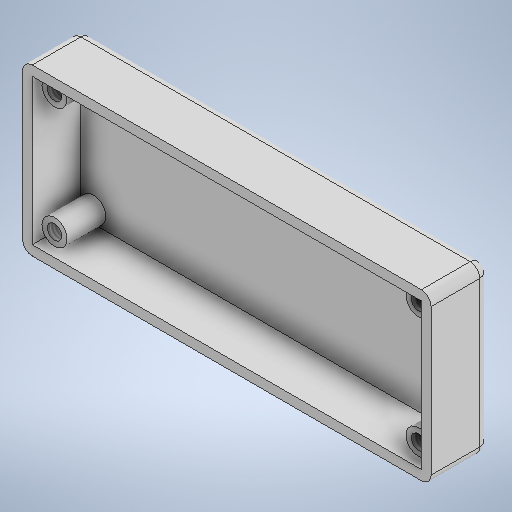
# Autodesk Inventor part: Bottom part of case
Saved by Autodesk Inventor 2025.2 (Build 292293000, 293)
## iProperties
Created: 2026-01-28
Part Number: Bottom part of case
Material: Generic
Document SubType Name: Modeling
Designer: seths
Density: 1 g/cm^3
Appearance: Default
Author: seths
Autodesk Inventor part; units mm, degrees
ref_plane "YZ Plane" through (0, 0, 0) normal (1, 0, 0) x (0, 1, 0)
ref_plane "XZ Plane" through (0, 0, 0) normal (0, 1, 0) x (-1, 0, 0)
ref_plane "XY Plane" through (0, 0, 0) normal (0, 0, 1) x (1, 0, 0)
sketch "Sketch1" plane through (0, 0, 0) normal (0, 0, 1) x (1, 0, 0)
  line L0 (0, 0) -> (-40, 0)
  line L1 (-40, 0) -> (-40, 15)
  line L2 (-40, 15) -> (0, 15)
  line L3 (0, 15) -> (0, 0)
  line L4 (1, -1) -> (-41, -1)
  line L5 (-41, -1) -> (-41, 16)
  line L6 (-41, 16) -> (1, 16)
  line L7 (1, 16) -> (1, -1)
  circle A0 centre (-1.293, 13.707) radius 0.75
  circle A1 centre (-1.293, 1.293) radius 0.75
  circle A2 centre (-38.707, 1.293) radius 0.75
  circle A3 centre (-38.707, 13.707) radius 0.75
  circle A4 centre (-38.707, 13.707) radius 1.293
  circle A5 centre (-38.707, 1.293) radius 1.293
  circle A6 centre (-1.293, 1.293) radius 1.293
  circle A7 centre (-1.293, 13.707) radius 1.293
  dimension "d0" = 40
  dimension "d1" = 15
  dimension "d2" = 42
  dimension "d3" = 17
  dimension "d4" = 1
  dimension "d6" = 1
  dimension "d7" = 1
  dimension "d8" = 1.5
  dimension "d9" = 1.5
  dimension "d10" = 1.293
  dimension "d11" = 1.293
  dimension "d12" = 1.293
  dimension "d13" = 1.293
  dimension "d14" = 1.5
  dimension "d15" = 1.293
  dimension "d16" = 1.293
  dimension "d17" = 1.5
  dimension "d18" = 1.293
  dimension "d19" = 1.293
  constraints: 16 end point, 8 centre point, 4 coincident, 4 parallel, 4 tangent, 2 horizontal, 2 perpendicular
  measures "d0" distance of L1.end L2.end
  measures "d1" distance of L0.end L1.end
  measures "d2" distance of L5.end L6.end
  measures "d3" distance of L4.end L5.end
  measures "d4" distance between parallel lines of L0 L4
  measures "d6" distance between parallel lines of L3 L7
  measures "d7" distance between parallel lines of L1 L5
  measures "d8" diameter of A3
  measures "d9" diameter of A2
  measures "d10" distance from line of L2 A3.centre
  measures "d11" distance from line of L1 A3.centre
  measures "d12" distance from line of L0 A2.centre
  measures "d13" distance from line of L1 A2.centre
  measures "d14" diameter of A1
  measures "d15" distance from line of L3 A1.centre
  measures "d16" distance from line of L0 A1.centre
  measures "d17" diameter of A0
  measures "d18" distance from line of L2 A0.centre
  measures "d19" distance from line of L3 A0.centre
extrude "Extrusion1" add sketch "Sketch1" along normal blind 6 contours L4 L5 L6 L7
extrude "Extrusion2" add sketch "Sketch1" along normal blind 1 contours L0 A6 L3 | L0 A5 L1 A4 L2 A7 L3 A6 | A6 | L0 L1 A5 | A5 | A7 L2 L3 | A7 | L1 L2 A4 | A4 | A0 | A1 | A2 | A3
extrude "Extrusion4" add sketch "Sketch1" along normal blind 5 contours A6 | A5 | A7 | A4
thread "Thread1" size "M1.6x0.35" class "6H" standard "ANSI Metric M Profile" full length
thread "Thread2" size "M1.6x0.35" class "6H" standard "ANSI Metric M Profile" full length
thread "Thread3" size "M1.6x0.35" class "6H" standard "ANSI Metric M Profile" full length
thread "Thread4" size "M1.6x0.35" class "6H" standard "ANSI Metric M Profile" full length
fillet "Fillet1" radius 1 8 edges at (1, 16, 3) (-41, 16, 3) (-41, -1, 3) (1, -1, 3) (1, 7.5, 0) (-20, 16, 0) (-20, -1, 0) (-41, 7.5, 0)
body "Solid1"
